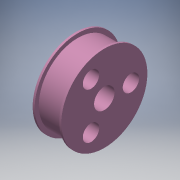
# Autodesk Inventor part: FoilCoil
Saved by Autodesk Inventor 2019 (Build 230136000, 136)
## iProperties
Created: 2017-01-18
Part Number: FoilCoil
Document SubType Name: Modeling
Designer: Administrator
Density: 1 g/cm^3
Mass: 1.78364 g
Surface Area: 14.31 cm^2
Volume: 1.78364 cm^3
Material: Generic
Appearance: Bubblegum
Author: Administrator
Autodesk Inventor part; units mm, degrees
ref_plane "YZ Plane" through (0, 0, 0) normal (1, 0, 0) x (0, 1, 0)
ref_plane "XZ Plane" through (0, 0, 0) normal (0, 1, 0) x (-1, 0, 0)
ref_plane "XY Plane" through (0, 0, 0) normal (0, 0, 1) x (1, 0, 0)
sketch "Sketch1" plane through (0, 0, 0) normal (0, 0, 1) x (1, 0, 0)
  line L0 (0, 0) -> (0, 9.5) construction
  line L1 (0, 9.5) -> (3, 9.5)
  line L2 (3, 9.5) -> (3, 10.5)
  line L3 (3, 10.5) -> (3.5, 10.5)
  line L4 (3.5, 10.5) -> (3.5, 0) construction
  line L5 (3.5, 0) -> (0, 0) construction
  line L6 (0, 2.5) -> (3.5, 2.5)
  line L7 (3.5, 2.5) -> (3.5, 10.5)
  line L8 (0, 9.5) -> (-3, 9.5)
  line L9 (-3, 9.5) -> (-3, 10.5)
  line L10 (-3, 10.5) -> (-3.5, 10.5)
  line L11 (-3.5, 10.5) -> (-3.5, 0) construction
  line L12 (0, 2.5) -> (-3.5, 2.5)
  line L13 (-3.5, 2.5) -> (-3.5, 10.5)
  dimension "d0" = 2.5
  dimension "d1" = 3
  dimension "d2" = 0.5
  dimension "d8" = 1
  dimension "d10" = 10.5
  constraints: 28 end point, 5 symmetric about line, 4 parallel, 3 point on line, 2 perpendicular, 1 collinear, 1 vertical, 1 other
  measures "d0" distance between parallel lines of L6 L5
  measures "d1" distance between parallel lines of L2 L0
  measures "d2" distance of L2.end L3.end
  measures "d8" distance between parallel lines of L3 L1
  measures "d10" distance between parallel lines of L3 L5
revolve "Revolution2" add sketch "Sketch1" angle 360 about axis through (3.5, 0, 0) along (-1, 0, 0)
sketch "Sketch2" plane through (3.5, 0, 0) normal (1, 0, 0) x (0, 0, -1)
  circle A0 centre (0, 0) radius 2.5 projected
  circle A1 centre (0, 6.5) radius 2
  dimension "d11" = 6.5
  dimension "d12" = 4
  constraints: 1 centre point
  measures "d11" distance of A1.centre A0.centre
  measures "d12" diameter of A1
extrude "Extrusion1" cut sketch "Sketch2" against normal through all contours A1
pattern_circular "Circular Pattern1" count 3 over 360 about axis through (1.5, 0, 0) along (1, 0, 0) of "Extrusion1"
body "Solid1"
